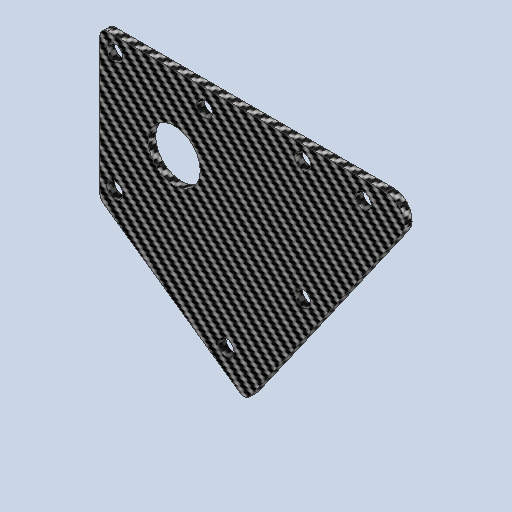
# Autodesk Inventor part: s_carbon_plate4
Saved by Autodesk Inventor 2022 (Build 260153000, 153)
## iProperties
Created: 2021-08-27
Part Number: s_carbon_plate4
Material: CFRP
Document SubType Name: Sheet Metal
Designer: Yuta Kage
Density: 1.43 g/cm^3
Sheet Metal Rule: Default_mm
Appearance: カーボンファイバー
Author: Yuta Kage
Autodesk Inventor part; units mm, degrees
ref_plane "YZ Plane" through (0, 0, 0) normal (1, 0, 0) x (0, 1, 0)
ref_plane "XZ Plane" through (0, 0, 0) normal (0, 1, 0) x (-1, 0, 0)
ref_plane "XY Plane" through (0, 0, 0) normal (0, 0, 1) x (1, 0, 0)
sketch "スケッチ1" plane through (0, 0, 0) normal (0, 0, 1) x (1, 0, 0)
  line L0 (-30, -20) -> (28.6, -20)
  line L1 (28.6, -20) -> (28.6, 20)
  line L2 (28.6, 20) -> (-30, 20)
  line L3 (-30, 20) -> (-30, -20)
  point P0 (0, 0)
  dimension "d1" = 40
  dimension "d28" = 30
  dimension "d29" = 28.6
  dimension "d32" = 20
  measures "d1" distance of L2.end L0.start
  measures "d28" distance from line of point (0, 0) L3
  measures "d29" distance from line of L1 point (0, 0)
  measures "d32" distance from line of point (0, 0) L2
extrude "プレート1" add sketch "スケッチ1" along normal blind 2
sketch "スケッチ2" plane through (0, 0, 2) normal (0, 0, 1) x (1, 0, 0)
  line L0 (-24, -5) -> (24.6, -5)
  line L1 (24.6, -5) -> (24.6, 5)
  line L2 (24.6, 5) -> (-24, 5)
  line L3 (-24, 5) -> (-24, -5)
  line L4 (-24, -5) -> (24.6, 5) construction
  line L5 (24.6, -5) -> (-24, 5) construction
  line L6 (28.6, -20) -> (-30, -20) projected
  line L7 (-30, -20) -> (-30, 20) projected
  line L8 (28.6, -20) -> (-30, -20) projected
  line L9 (28.6, 20) -> (28.6, -20) projected
  line L10 (-30, 20) -> (28.6, 20) projected
  circle A0 centre (-10, 0) radius 7
  point P0 (0.3, 0)
  point P1 (0.3, 0)
  point P2 (0.3, 0)
  point P3 (0, 0)
  dimension "GapSize" = 2
  dimension "d3" = 48.6
  dimension "d5" = 10
  dimension "d8" = 20
  dimension "d16" = 14
  dimension "d30" = 20
  dimension "d31" = 14
  constraints: 12 end point, 4 midpoint, 2 parallel, 1 centre point, 1 coincident, 1 horizontal, 1 horizontal alignment, 1 perpendicular
  measures "d3" distance of L1.end L2.end
  measures "d5" distance of L0.end L1.end
  measures "d8" distance from line of L6 point (0.3, 0)
  measures "d16" diameter of A0
  measures "d30" distance from line of L7 A0.centre
  measures "d31" distance from line of L3 A0.centre
extrude "押し出し1" cut sketch "スケッチ2" against normal blind 10 contours A0 L2 L0 | L0 A0 | A0 L2
sketch "スケッチ3" plane through (0, 0, 2) normal (0, 0, 1) x (1, 0, 0)
  line L0 (-30, 20) -> (28.6, 20) projected
  line L1 (-30, -20) -> (-30, 20) projected
  line L2 (28.6, -20) -> (-30, -20) projected
  line L3 (28.6, 20) -> (28.6, -20) projected
  line L4 (24.6, 16) -> (-26, 16)
  line L5 (-26, 16) -> (-26, -16)
  line L6 (-26, -16) -> (24.6, -16)
  line L7 (24.6, -16) -> (24.6, 16)
  point P0 (0, 0)
  dimension "d19" = 4
  constraints: 8 end point, 3 other
  measures "d19" distance between parallel lines of L0 L4
hole "穴2" at (-26, 16, 2) at (-26, -16, 2) at (24.6, 16, 2) at (24.6, -16, 2) direction (0, 0, -1) diameter 4.3 end through all clearance for "Socket Head Cap Screw" size "M4" standard "Ansi Metric M Profile"
sketch "スケッチ4" plane through (0, 0, 2) normal (0, 0, 1) x (1, 0, 0)
  line L0 (-30, -20) -> (28.6, -20)
  line L1 (28.6, -20) -> (56.6083, 20)
  line L2 (28.6, 20) -> (28.6, -20)
  line L3 (28.6, 20) -> (56.6083, 20)
  line L4 (-30, -20) -> (9.3212, -47.533)
  line L5 (28.6, -20) -> (9.3212, -47.533)
  point P0 (0, 0)
  dimension "d33" = 35
  dimension "d34" = 35
  measures "d33" angle of L1 L2
  measures "d34" angle of L0 L4
sheet face with bend "面2" sketch "スケッチ4" thickness 2 toward (0, 0, -1) bend radius 2
bend "曲げ1"
sketch "スケッチ5" plane through (0, 0, 2) normal (0, 0, 1) x (1, 0, 0)
  line L0 (-30, -20) -> (9.3212, -47.533) projected
  line L1 (9.3212, -47.533) -> (56.6083, 20) projected
  line L2 (56.6083, 20) -> (-30, 20) projected
  point P0 (0, 0)
  point P1 (3.9976, -37.7015)
  point P2 (40.8995, 15)
  point P3 (-1.8276, 15)
  dimension "d40" = 5
  dimension "d41" = 10
  dimension "d42" = 10
  dimension "d43" = 5
  dimension "d44" = 5
  dimension "d45" = 45
  measures "d40" distance from line of L0 point (3.998, -37.701)
  measures "d41" distance from line of L1 point (3.998, -37.701)
  measures "d42" distance from line of L1 point (40.9, 15)
  measures "d43" distance from line of L2 point (40.9, 15)
  measures "d44" distance from line of L2 point (-1.828, 15)
  measures "d45" distance from line of L1 point (-1.828, 15)
hole "穴3" at (3.9976, -37.7015, 2) at (40.8995, 15, 2) at (-1.8276, 15, 2) direction (0, 0, -1) diameter 4.3 end through all
fillet "フィレット1" radius 2 3 edges at (-30, 20, 1) (-30, -20, 1) (9.3212, -47.533, 1)
fillet "フィレット2" radius 5 1 edges at (56.6083, 20, 1)
equation "\"GapSize\" = Thickness"
equation "\"d42\" = d41"
equation "\"d43\" = d40"
equation "\"d44\" = d40"
equation "\"d51\" = Thickness"
equation "\"d2\" = Thickness"
equation "\"d35\" = BendRadius"
equation "\"d36\" = BendReliefWidth"
equation "\"d38\" = MinimumRemnant"
equation "\"d37\" = BendReliefDepth"
equation "\"d39\" = TransitionRadius"
equation "\"BendRadius\" = Thickness"
equation "\"BendReliefWidth\" = Thickness"
equation "\"BendReliefDepth\" = 0.5 * Thickness"
equation "\"CornerReliefSize\" = 4 * Thickness"
equation "\"MinimumRemnant\" = 2 * Thickness"
equation "\"TransitionRadius\" = BendRadius"
equation "\"JacobiRadiusSize\" = BendRadius"
equation "\"Thickness\" = 2"
